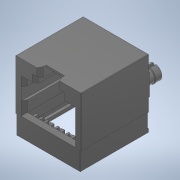
# Autodesk Inventor part: RJ45 Main Insert
Saved by Autodesk Inventor 2020.1 (Build 241239000, 239)
## iProperties
Created: 2019-12-05
Part Number: RJ45 Main Insert
Material: PBT Plastic
Document SubType Name: Modeling
Designer: S. Lee
Mass: 2.00676 g
Surface Area: 24.163 cm^2
Volume: 1.53188 cm^3
Density: 1.31 g/cm^3
Appearance: Smooth - Black
Author: S. Lee
Autodesk Inventor part; units mm, degrees
ref_plane "YZ Plane" through (0, 0, 0) normal (1, 0, 0) x (0, 1, 0)
ref_plane "XZ Plane" through (0, 0, 0) normal (0, 1, 0) x (-1, 0, 0)
ref_plane "XY Plane" through (0, 0, 0) normal (0, 0, 1) x (1, 0, 0)
sketch "Sketch1" plane through (0, 0, 0) normal (0, 0, 1) x (1, 0, 0)
  line L0 (-7.75, 8.125) -> (7.75, 8.125)
  line L1 (7.75, 8.125) -> (7.75, -3.775)
  line L2 (7.54, -8.125) -> (-7.54, -8.125)
  line L3 (-7.75, -3.775) -> (-7.75, 8.125)
  line L4 (-7.75, -3.775) -> (-7.54, -3.775)
  line L5 (-7.54, -3.775) -> (-7.54, -8.125)
  line L6 (7.75, -3.775) -> (7.54, -3.775)
  line L7 (7.54, -3.775) -> (7.54, -8.125)
  line L8 (0, -11.375) -> (0, 11.375) construction
  line L9 (-10.85, 0) -> (10.85, 0) construction
  dimension "d5" = 16.25
  dimension "d6" = 15.5
  dimension "d7" = 15.08
  dimension "d8" = 4.35
  constraints: 16 end point, 3 horizontal, 3 perpendicular, 2 parallel, 1 point on line, 3 other
  measures "d5" distance between parallel lines of L2 L0
  measures "d6" distance between parallel lines of L1 L3
  measures "d7" distance between parallel lines of L7 L5
  measures "d8" distance between parallel lines of L2 L4
extrude "Extrusion1" add sketch "Sketch1" against normal blind 16
sketch "Sketch2" plane through (0, 0, 0) normal (0, 0, 1) x (1, 0, 0)
  line L0 (5.925, -3.125) -> (-5.925, -3.125)
  line L1 (3.32, 4.125) -> (3.32, 5.825)
  line L2 (3.32, 5.825) -> (-3.32, 5.825)
  line L3 (-3.32, 5.825) -> (-3.32, 4.125)
  line L4 (-5.925, 4.125) -> (-3.32, 4.125)
  line L5 (3.32, 4.125) -> (5.925, 4.125)
  line L6 (-5.925, 2.325) -> (-6.425, 2.325)
  line L7 (-6.425, 2.325) -> (-6.425, -0.525)
  line L8 (-6.425, -0.525) -> (-5.925, -0.525)
  line L9 (5.925, 2.325) -> (6.425, 2.325)
  line L10 (6.425, 2.325) -> (6.425, -0.525)
  line L11 (6.425, -0.525) -> (5.925, -0.525)
  line L12 (-5.925, -3.125) -> (-5.925, -0.525)
  line L13 (-5.925, 2.325) -> (-5.925, 4.125)
  line L14 (5.925, 4.125) -> (5.925, 2.325)
  line L15 (5.925, -0.525) -> (5.925, -3.125)
  line L16 (0, -11.375) -> (0, 11.375) construction
  line L17 (-7.54, -8.125) -> (7.54, -8.125) construction
  point P0 (0, 0)
  dimension "d12" = 6.64
  dimension "d13" = 12.85
  dimension "d14" = 11.85
  dimension "d15" = 7.25
  dimension "d16" = 2.85
  dimension "d17" = 2.6
  dimension "d18" = 8.95
  dimension "d19" = 5
  constraints: 32 end point, 9 parallel, 6 perpendicular, 4 horizontal, 3 collinear, 2 point on line, 3 other
  measures "d12" distance between parallel lines of L1 L3
  measures "d13" distance between parallel lines of L10 L7
  measures "d14" distance between parallel lines of L15 L12
  measures "d15" distance between parallel lines of L0 L4
  measures "d16" distance between parallel lines of L8 L6
  measures "d17" distance between parallel lines of L0 L8
  measures "d18" distance between parallel lines of L0 L2
  measures "d19" distance between parallel lines of L17 L0
extrude "Extrusion2" cut sketch "Sketch2" against normal blind 12.7
sketch "Sketch3" plane through (0, 0, 0) normal (0, 0, 1) x (1, 0, 0)
  line L0 (-7.75, 8.125) -> (7.75, 8.125) construction
  line L1 (-3.32, 5.825) -> (3.32, 5.825) construction
  line L2 (-2.18, 8.125) -> (2.18, 8.125)
  line L3 (2.18, 8.125) -> (2.18, 5.825)
  line L4 (2.18, 5.825) -> (-2.18, 5.825)
  line L5 (-2.18, 5.825) -> (-2.18, 8.125)
  line L6 (0, -11.375) -> (0, 11.375) construction
  point P0 (0, 0)
  dimension "d22" = 4.36
  constraints: 8 end point, 2 parallel, 2 point on line, 1 horizontal, 1 perpendicular, 1 other
  measures "d22" distance of L3.end L4.end
extrude "Extrusion3" cut sketch "Sketch3" against normal blind 1.65
chamfer "Chamfer1" distance 0.5 distance2 1 1 edges at (0, -3.125, 0) measured on face at (0, -3.625, 0)
chamfer "Chamfer2" distance 0.5 distance2 1 2 edges at (-5.925, -3.375, 0) (-5.925, -1.825, 0) measured on face at (-6.425, -1.825, 0) measured on face at (-6.425, -3.375, 0)
chamfer "Chamfer3" distance 0.5 distance2 1 1 edges at (-5.925, 3.225, 0) measured on face at (-6.425, 3.225, 0)
chamfer "Chamfer4" distance 0.5 distance2 1 2 edges at (-6.175, 4.125, 0) (-4.6225, 4.125, 0) measured on face at (-4.6225, 4.625, 0) measured on face at (-6.175, 4.625, 0)
chamfer "Chamfer5" distance 0.5 distance2 1 1 edges at (-3.32, 5.225, 0) measured on face at (-3.82, 5.225, 0)
chamfer "Chamfer6" distance 0.5 distance2 1 2 edges at (-3.57, 5.825, 0) (-2.75, 5.825, 0) measured on face at (-2.75, 6.325, 0) measured on face at (-3.57, 6.325, 0)
chamfer "Chamfer7" distance 0.5 distance2 1 1 edges at (-2.18, 7.225, 0) measured on face at (-2.68, 7.225, 0)
chamfer "Chamfer8" distance 0.5 distance2 1 1 edges at (2.18, 6.975, 0) measured on face at (2.68, 6.975, 0)
chamfer "Chamfer9" distance 0.5 distance2 1 1 edges at (3, 5.825, 0)
chamfer "Chamfer10" distance 0.5 distance2 1 2 edges at (3.32, 6.0749, 0) (3.32, 4.975, 0) measured on face at (3.82, 6.0749, 0) measured on face at (3.82, 4.975, 0)
chamfer "Chamfer11" distance 0.5 distance2 1 1 edges at (4.8725, 4.125, 0) measured on face at (4.8725, 4.625, 0)
chamfer "Chamfer12" distance 0.5 distance2 1 2 edges at (5.925, 4.375, 0) (5.925, 3.225, 0) measured on face at (6.425, 3.225, 0) measured on face at (6.425, 4.375, 0)
chamfer "Chamfer13" distance 0.5 distance2 1 2 edges at (5.925, -1.825, 0) (5.925, -3.375, 0) measured on face at (6.425, -3.375, 0) measured on face at (6.425, -1.825, 0)
sketch "Sketch4" plane through (0, 0, -1.65) normal (0, 0, 1) x (1, 0, 0)
  line L0 (2.18, 5.825) -> (-2.18, 5.825) construction
  line L1 (-2.18, 7.695) -> (2.18, 7.695)
  line L2 (2.18, 7.695) -> (2.18, 5.825)
  line L3 (2.18, 5.825) -> (-2.18, 5.825)
  line L4 (-2.18, 5.825) -> (-2.18, 7.695)
  line L5 (-2.18, 5.825) -> (-2.18, 8.125) construction
  line L6 (2.18, 8.125) -> (2.18, 5.825) construction
  point P0 (0, 0)
  dimension "d64" = 1.87
  constraints: 8 end point, 2 collinear, 2 parallel, 1 horizontal, 1 perpendicular, 1 point on line
  measures "d64" distance between parallel lines of L0 L1
extrude "Extrusion4" cut sketch "Sketch4" against normal blind 1
sketch "Sketch5" plane through (0, 0, -2.65) normal (0, 0, 1) x (1, 0, 0)
  line L0 (2.18, 5.825) -> (-2.18, 5.825) construction
  line L1 (-2.18, 5.825) -> (2.18, 5.825)
  line L2 (2.18, 5.825) -> (2.18, 7.375)
  line L3 (2.18, 7.375) -> (-2.18, 7.375)
  line L4 (-2.18, 7.375) -> (-2.18, 5.825)
  line L5 (-2.18, 5.825) -> (-2.18, 7.695) construction
  line L6 (2.18, 7.695) -> (2.18, 5.825) construction
  point P0 (0, 0)
  dimension "d67" = 1.55
  constraints: 8 end point, 2 collinear, 2 parallel, 1 horizontal, 1 perpendicular, 1 point on line
  measures "d67" distance of L2.end L1.end
extrude "Extrusion5" cut sketch "Sketch5" against normal blind 3
chamfer "Chamfer14" distance 0.32 distance2 0.95 1 edges at (0, 7.375, -2.65) measured on face at (0, 7.475, -2.65)
sketch "Sketch6" plane through (0, 0, -16) normal (0, 0, -1) x (-1, 0, 0)
  line L0 (3.99, 7.025) -> (3.99, -0.65)
  line L1 (-3.99, -0.65) -> (-3.99, 7.025)
  line L2 (6.425, -8.125) -> (-6.425, -8.125)
  line L3 (-6.425, -0.65) -> (-3.99, -0.65)
  line L4 (3.99, -0.65) -> (6.425, -0.65)
  line L5 (0, -11.375) -> (0, 11.375) construction
  line L6 (7.75, 8.125) -> (-7.75, 8.125) construction
  line L7 (3.99, 7.025) -> (-3.99, 7.025)
  line L8 (-6.425, -5.925) -> (-7.06, -5.925)
  line L9 (-7.06, -5.925) -> (-7.06, -7.325)
  line L10 (-7.06, -7.325) -> (-6.425, -7.325)
  line L11 (6.425, -5.925) -> (7.06, -5.925)
  line L12 (7.06, -5.925) -> (7.06, -7.325)
  line L13 (7.06, -7.325) -> (6.425, -7.325)
  line L14 (-6.425, -8.125) -> (-6.425, -7.325)
  line L15 (-6.425, -5.925) -> (-6.425, -0.65)
  line L16 (6.425, -0.65) -> (6.425, -5.925)
  line L17 (6.425, -7.325) -> (6.425, -8.125)
  line L18 (-7.54, -8.125) -> (7.54, -8.125) construction
  point P0 (0, 0)
  dimension "d75" = 7.98
  dimension "d81" = 12.85
  dimension "d82" = 14.12
  dimension "d83" = 1.4
  dimension "d84" = 0.8
  dimension "d85" = 7.675
  dimension "d86" = 1.1
  constraints: 32 end point, 9 parallel, 6 perpendicular, 4 collinear, 4 horizontal, 2 point on line, 3 other
  measures "d75" distance between parallel lines of L0 L1
  measures "d81" distance between parallel lines of L16 L15
  measures "d82" distance between parallel lines of L12 L9
  measures "d83" distance between parallel lines of L10 L8
  measures "d84" distance between parallel lines of L2 L10
  measures "d85" distance between parallel lines of L3 L7
  measures "d86" distance between parallel lines of L6 L7
extrude "Extrusion6" cut sketch "Sketch6" against normal blind 1.2
sketch "Sketch8" plane through (0, 0, -14.8) normal (0, 0, -1) x (-1, 0, 0)
  line L0 (6.425, -8.125) -> (-6.425, -8.125) projected
  line L1 (-6.425, -8.125) -> (-6.425, -7.325) projected
  line L2 (-7.06, -7.325) -> (-7.06, -5.925) projected
  line L3 (-6.425, -5.925) -> (-6.425, -0.65) projected
  line L4 (-7.06, -5.925) -> (-6.425, -5.925) projected
  line L5 (6.425, -5.925) -> (7.06, -5.925) projected
  line L6 (6.425, -0.65) -> (6.425, -5.925) projected
  line L7 (7.06, -5.925) -> (7.06, -7.325) projected
  line L8 (6.425, -7.325) -> (6.425, -8.125) projected
  line L9 (-6.425, -7.325) -> (-7.06, -7.325) projected
  line L10 (7.06, -7.325) -> (6.425, -7.325) projected
  line L11 (-6.425, -3.125) -> (6.425, -3.125)
  point P0 (0, 0)
  dimension "d87" = 5
  constraints: 2 end point, 2 point on line, 1 perpendicular
  measures "d87" distance between parallel lines of L0 L11
extrude "Extrusion7" cut sketch "Sketch8" against normal blind 10.9
sketch "Sketch9" plane through (0, 0, -3.9) normal (0, 0, -1) x (-1, 0, 0)
  line L0 (-5.925, -3.125) -> (5.925, -3.125) projected
  line L1 (-7.06, -5.925) -> (-6.425, -5.925) projected
  line L2 (-7.06, -7.325) -> (-7.06, -5.925) projected
  line L3 (-6.425, -7.325) -> (-7.06, -7.325) projected
  line L4 (-6.425, -8.125) -> (-6.425, -7.325) projected
  line L5 (6.425, -8.125) -> (-6.425, -8.125) projected
  line L6 (6.425, -7.325) -> (6.425, -8.125) projected
  line L7 (7.06, -7.325) -> (6.425, -7.325) projected
  line L8 (7.06, -5.925) -> (7.06, -7.325) projected
  line L9 (6.425, -5.925) -> (7.06, -5.925) projected
  line L10 (6.425, -3.125) -> (6.425, -5.925) projected
  line L11 (5.925, -3.125) -> (6.425, -3.125) projected
  line L12 (-5.925, -3.125) -> (5.925, -3.125) projected
  line L13 (-6.425, -3.125) -> (-5.925, -3.125) projected
  line L14 (-6.425, -5.925) -> (-6.425, -3.125) projected
  line L15 (-6.425, -7.325) -> (6.425, -7.325)
  point P0 (0, 0)
  point P1 (5.925, -3.125)
  constraints: 2 end point, 1 horizontal
extrude "Extrusion8" cut sketch "Sketch9" against normal blind 2.9 contours L0 L11 L10 L9 L8 L7 L15 L3 L2 L1 L14 L13
sketch "Sketch10" plane through (0, 0, -14.8) normal (0, 0, -1) x (-1, 0, 0)
  line L0 (-3.99, 7.025) -> (3.99, 7.025) projected
  line L1 (3.99, 7.025) -> (3.99, -0.65) projected
  line L2 (-3.99, 7.025) -> (3.99, 7.025)
  line L3 (3.99, 7.025) -> (3.99, 5.825)
  line L4 (3.99, 5.825) -> (-3.99, 5.825)
  line L5 (-3.99, 5.825) -> (-3.99, 7.025)
  point P0 (0, 0)
  dimension "d92" = 1.2
  constraints: 8 end point, 2 parallel, 1 horizontal, 1 perpendicular, 1 point on line
  measures "d92" distance between parallel lines of L4 L0
extrude "Extrusion9" cut sketch "Sketch10" against normal blind 11.2
sketch "Sketch11" plane through (0, 0, -12.7) normal (0, 0, 1) x (1, 0, 0)
  line L0 (6.425, -3.125) -> (-6.425, -3.125) projected
  line L1 (-4.67, -3.125) -> (-4.22, -3.125)
  line L2 (-4.22, -3.125) -> (-4.22, 1.225)
  line L3 (-4.22, 1.225) -> (-4.67, 1.225)
  line L4 (-4.67, 1.225) -> (-4.67, -3.125)
  line L5 (-7.75, -3.775) -> (-7.75, 8.125) projected
  line L6 (-3.4, -3.125) -> (-2.95, -3.125)
  line L7 (-2.95, -3.125) -> (-2.95, 1.225)
  line L8 (-2.95, 1.225) -> (-3.4, 1.225)
  line L9 (-3.4, 1.225) -> (-3.4, -3.125)
  line L10 (-2.13, -3.125) -> (-1.68, -3.125)
  line L11 (-1.68, -3.125) -> (-1.68, 1.225)
  line L12 (-1.68, 1.225) -> (-2.13, 1.225)
  line L13 (-2.13, 1.225) -> (-2.13, -3.125)
  line L14 (-0.86, -3.125) -> (-0.41, -3.125)
  line L15 (-0.41, -3.125) -> (-0.41, 1.225)
  line L16 (-0.41, 1.225) -> (-0.86, 1.225)
  line L17 (-0.86, 1.225) -> (-0.86, -3.125)
  line L18 (0.41, -3.125) -> (0.86, -3.125)
  line L19 (0.86, -3.125) -> (0.86, 1.225)
  line L20 (0.86, 1.225) -> (0.41, 1.225)
  line L21 (0.41, 1.225) -> (0.41, -3.125)
  line L22 (1.68, -3.125) -> (2.13, -3.125)
  line L23 (2.13, -3.125) -> (2.13, 1.225)
  line L24 (2.13, 1.225) -> (1.68, 1.225)
  line L25 (1.68, 1.225) -> (1.68, -3.125)
  line L26 (2.95, -3.125) -> (3.4, -3.125)
  line L27 (3.4, -3.125) -> (3.4, 1.225)
  line L28 (3.4, 1.225) -> (2.95, 1.225)
  line L29 (2.95, 1.225) -> (2.95, -3.125)
  line L30 (4.22, -3.125) -> (4.67, -3.125)
  line L31 (4.67, -3.125) -> (4.67, 1.225)
  line L32 (4.67, 1.225) -> (4.22, 1.225)
  line L33 (4.22, 1.225) -> (4.22, -3.125)
  point P0 (0, 0)
  dimension "d95" = 0.45
  dimension "d96" = 4.35
  dimension "d97" = 3.08
  dimension "d100" = 1.27
  constraints: 64 end point, 2 horizontal, 2 parallel, 1 perpendicular, 1 point on line, 56 other
  measures "d95" distance of L3.end L2.end
  measures "d96" distance of L1.end L2.end
  measures "d97" distance between parallel lines of L5 L4
  measures "d100" distance of L1.start L6.start
extrude "Extrusion10" cut sketch "Sketch11" against normal up to surface (2.1 mm away)
chamfer "Chamfer15" distance 0.9 distance2 2.1 1 edges at (3.81, -3.125, -14.8) measured on face at (3.81, -2.625, -14.8)
chamfer "Chamfer16" distance 0.9 distance2 2.1 1 edges at (2.54, -3.125, -14.8) measured on face at (2.54, -2.625, -14.8)
chamfer "Chamfer17" distance 0.9 distance2 2.1 1 edges at (1.27, -3.125, -14.8) measured on face at (1.27, -2.625, -14.8)
chamfer "Chamfer18" distance 0.9 distance2 2.1 1 edges at (0, -3.125, -14.8) measured on face at (0, -2.625, -14.8)
chamfer "Chamfer19" distance 0.9 distance2 2.1 1 edges at (-1.27, -3.125, -14.8) measured on face at (-1.27, -2.625, -14.8)
chamfer "Chamfer20" distance 0.9 distance2 2.1 1 edges at (-2.54, -3.125, -14.8) measured on face at (-2.54, -2.625, -14.8)
chamfer "Chamfer21" distance 0.9 distance2 2.1 1 edges at (-3.81, -3.125, -14.8) measured on face at (-3.81, -2.625, -14.8)
chamfer "Chamfer22" distance 0.9 distance2 2.1 1 edges at (1.905, 1.225, -14.8) measured on face at (1.905, 1.725, -14.8)
chamfer "Chamfer23" distance 0.9 distance2 2.1 1 edges at (3.175, 1.225, -14.8) measured on face at (3.175, 1.725, -14.8)
chamfer "Chamfer24" distance 0.9 distance2 2.1 1 edges at (0.635, 1.225, -14.8) measured on face at (0.635, 1.725, -14.8)
chamfer "Chamfer25" distance 0.9 distance2 2.1 1 edges at (-0.635, 1.225, -14.8) measured on face at (-0.635, 1.725, -14.8)
chamfer "Chamfer26" distance 0.9 distance2 2.1 1 edges at (-1.905, 1.225, -14.8) measured on face at (-1.905, 1.725, -14.8)
chamfer "Chamfer27" distance 0.9 distance2 2.1 1 edges at (-3.175, 1.225, -14.8) measured on face at (-3.175, 1.725, -14.8)
sketch "Sketch12" plane through (-4.67, -3.125, -12.7) normal (1, 0, 0) x (0, 0, -1)
  line L0 (0, 4.35) -> (2.1, 5.25) projected
  line L1 (2.1, 5.25) -> (2.1, 2.475)
  line L2 (2.1, 2.475) -> (0, 2.475)
  line L3 (0, 2.475) -> (0, 4.35)
  line L4 (3.3, 2.475) -> (2.1, 2.475) construction
  point P0 (-12.7, 3.125)
  constraints: 6 end point, 2 perpendicular, 1 collinear, 1 vertical
extrude "Extrusion11" cut sketch "Sketch12" along normal up to surface (0.45 mm away)
sketch "Sketch13" plane through (4.22, -0.65, -14.8) normal (1, 0, 0) x (0, 0, -1)
  line L0 (-2.1, 1.875) -> (0, 2.775) projected
  line L1 (1.2, 0) -> (0, 0) projected
  line L2 (0, 2.775) -> (0, 0)
  line L3 (0, 0) -> (-2.1, 0)
  line L4 (-2.1, 1.875) -> (-2.1, -2.475) projected
  line L5 (-2.1, 0) -> (-2.1, 1.875)
  point P0 (-14.8, 0.65)
  constraints: 6 end point, 2 perpendicular, 1 collinear
extrude "Extrusion12" cut sketch "Sketch13" along normal up to surface (0.45 mm away)
sketch "Sketch14" plane through (0, 0, -16) normal (0, 0, -1) x (-1, 0, 0)
  line L0 (-7.75, -3.775) -> (-7.75, 8.125) construction
  line L1 (-7.75, 4.3) -> (-5.85, 4.3)
  line L2 (-5.85, 4.3) -> (-5.85, -0.65)
  line L3 (-5.85, -0.65) -> (-7.75, -0.65)
  line L4 (-7.75, -0.65) -> (-7.75, 4.3)
  line L5 (-6.425, -0.65) -> (-3.99, -0.65) construction
  arc A0 (-5.85, 0.2558) -> (-5.85, 3.3942) centre (-5.715, 1.825) ccw
  point P0 (0, 0)
  dimension "d150" = 1.9
  dimension "d151" = 4.95
  dimension "d154" = 2.475
  dimension "d157" = 1.575
  dimension "d158" = 2.035
  constraints: 6 end point, 2 horizontal, 2 point on circle, 1 centre point, 1 collinear, 1 parallel, 1 point on line, 1 vertical, 5 other
  measures "d150" distance of L3.start L3.end
  measures "d151" distance of L1.end L3.start
  measures "d154" distance from line of L1 A0.centre
  measures "d157" radius of A0
  measures "d158" distance from line of L0 A0.centre
extrude "Extrusion13" add sketch "Sketch14" along normal blind 0.2
sketch "Sketch15" plane through (0, 0, -16.2) normal (0, 0, -1) x (-1, 0, 0)
  arc A0 (-5.85, 0.2558) -> (-5.85, 3.3942) centre (-5.715, 1.825) ccw projected
  circle A1 centre (-5.715, 1.825) radius 1.575
  line L0 (-6.065, 3.3606) -> (-6.065, 0.2894)
  line L1 (-5.365, 0.2894) -> (-5.365, 3.3606)
  line L2 (-5.715, 1.825) -> (-5.715, 3.4) construction
  point P0 (0, 0)
  dimension "d159" = 0.7
  constraints: 6 end point, 5 point on circle, 2 vertical, 1 centre point, 1 coincident, 1 concentric, 1 parallel, 1 other
  measures "d159" distance between parallel lines of L1 L0
extrude "Extrusion14" add sketch "Sketch15" along normal blind 1.65 contours L1 A0 | A1 L0
sketch "Sketch16" plane through (0, 0, -17.85) normal (0, 0, -1) x (-1, 0, 0)
  line L0 (-5.365, 3.3606) -> (-5.365, 0.2894) construction
  line L1 (-6.065, 0.2894) -> (-6.065, 3.3606) construction
  circle A0 centre (-5.715, 1.825) radius 1.725
  line L2 (-6.065, 3.5141) -> (-6.065, 0.1359)
  line L3 (-5.365, 3.5141) -> (-5.365, 0.1359)
  arc A1 (-6.065, 3.3606) -> (-6.065, 0.2894) centre (-5.715, 1.825) ccw projected
  point P0 (0, 0)
  dimension "d162" = 3.45
  constraints: 4 end point, 4 point on circle, 2 collinear, 1 centre point, 1 coincident, 1 vertical
  measures "d162" diameter of A0
extrude "Extrusion15" add sketch "Sketch16" along normal blind 1.85 contours A0 L3 | L2 A1 A0 | L2 A1
chamfer "Chamfer28" distance 0.15 angle 45 2 edges at (7.44, 1.825, -17.85) (3.99, 1.825, -17.85)
chamfer "Chamfer29" distance 0.6 distance2 0.3 1 edges at (7.44, 1.825, -19.7) measured on face at (6.94, 1.825, -19.7)
chamfer "Chamfer30" distance 0.6 distance2 0.3 1 edges at (3.99, 1.825, -19.7) measured on face at (4.49, 1.825, -19.7)
sketch "Sketch17" plane through (0, 0, -16) normal (0, 0, -1) x (-1, 0, 0)
  circle A0 centre (-6.3, 6.975) radius 0.45
  line L0 (7.75, 8.125) -> (-7.75, 8.125) construction
  line L1 (-7.75, 8.125) -> (-7.75, 4.3) construction
  line L2 (-6.425, -8.125) -> (-6.425, -7.325) projected
  line L3 (-7.54, -3.775) -> (-7.54, -8.125) projected
  line L4 (-6.425, -7.325) -> (-7.54, -7.325)
  line L5 (-7.54, -7.325) -> (-7.54, -8.125)
  line L6 (-7.54, -8.125) -> (-6.425, -8.125)
  line L7 (-6.425, -8.125) -> (-6.425, -7.325)
  point P0 (0, 0)
  dimension "d174" = 0.9
  dimension "d175" = 1.15
  dimension "d176" = 1.45
  constraints: 8 end point, 2 parallel, 1 centre point, 1 horizontal, 1 perpendicular
  measures "d174" diameter of A0
  measures "d175" distance from line of L0 A0.centre
  measures "d176" distance from line of L1 A0.centre
extrude "Extrusion16" add sketch "Sketch17" along normal blind 0.2
mirror "Mirror1" about plane through (0, 0, 0) normal (1, 0, 0) of "Extrusion16", "Extrusion15", "Extrusion14", "Extrusion13", "Chamfer28", "Chamfer29", "Chamfer30"
sketch "Sketch19" plane through (0, 0, -1) normal (0, 0, -1) x (-1, 0, 0)
  line L0 (6.425, -7.325) -> (-6.425, -7.325) construction
  line L1 (-6.425, -8.125) -> (-6.425, -7.325) construction
  line L2 (6.425, -8.125) -> (-6.425, -8.125) construction
  line L3 (6.425, -7.325) -> (6.425, -8.125) construction
  line L4 (-4.67, 1.225) -> (-4.67, -3.125) construction
  line L5 (-4.22, -3.125) -> (-4.22, 1.225) construction
  line L6 (-4.22, -7.325) -> (4.22, -7.325)
  line L7 (4.22, -7.325) -> (4.22, -5.825)
  line L8 (4.22, -5.825) -> (-4.22, -5.825)
  line L9 (-4.22, -5.825) -> (-4.22, -7.325)
  line L10 (-4.67, -3.125) -> (-4.22, -3.125)
  line L11 (-4.22, -3.125) -> (-4.22, -5.125)
  line L12 (-4.22, -5.125) -> (-4.67, -5.125)
  line L13 (-4.67, -5.125) -> (-4.67, -3.125)
  line L14 (0, -11.375) -> (0, 11.375) construction
  line L15 (-3.4, -3.125) -> (-2.95, -3.125)
  line L16 (-2.95, -3.125) -> (-2.95, -5.125)
  line L17 (-2.95, -5.125) -> (-3.4, -5.125)
  line L18 (-3.4, -5.125) -> (-3.4, -3.125)
  line L19 (-2.13, -3.125) -> (-1.68, -3.125)
  line L20 (-1.68, -3.125) -> (-1.68, -5.125)
  line L21 (-1.68, -5.125) -> (-2.13, -5.125)
  line L22 (-2.13, -5.125) -> (-2.13, -3.125)
  line L23 (-0.86, -3.125) -> (-0.41, -3.125)
  line L24 (-0.41, -3.125) -> (-0.41, -5.125)
  line L25 (-0.41, -5.125) -> (-0.86, -5.125)
  line L26 (-0.86, -5.125) -> (-0.86, -3.125)
  line L27 (0.41, -3.125) -> (0.86, -3.125)
  line L28 (0.86, -3.125) -> (0.86, -5.125)
  line L29 (0.86, -5.125) -> (0.41, -5.125)
  line L30 (0.41, -5.125) -> (0.41, -3.125)
  line L31 (1.68, -3.125) -> (2.13, -3.125)
  line L32 (2.13, -3.125) -> (2.13, -5.125)
  line L33 (2.13, -5.125) -> (1.68, -5.125)
  line L34 (1.68, -5.125) -> (1.68, -3.125)
  line L35 (2.95, -3.125) -> (3.4, -3.125)
  line L36 (3.4, -3.125) -> (3.4, -5.125)
  line L37 (3.4, -5.125) -> (2.95, -5.125)
  line L38 (2.95, -5.125) -> (2.95, -3.125)
  line L39 (4.22, -3.125) -> (4.67, -3.125)
  line L40 (4.67, -3.125) -> (4.67, -5.125)
  line L41 (4.67, -5.125) -> (4.22, -5.125)
  line L42 (4.22, -5.125) -> (4.22, -3.125)
  point P0 (0, 0)
  dimension "d179" = 1.5
  dimension "d180" = 8.44
  dimension "d181" = 2
  dimension "d184" = 1.27
  constraints: 72 end point, 4 parallel, 3 horizontal, 2 perpendicular, 1 collinear, 1 point on line, 57 other
  measures "d179" distance of L8.end L6.start
  measures "d180" distance between parallel lines of L7 L9
  measures "d181" distance between parallel lines of L12 L10
  measures "d184" distance of L4.end L15.start
extrude "Extrusion17" add sketch "Sketch19" along normal blind 0.8
sketch "Sketch20" plane through (0, 0, -1) normal (0, 0, -1) x (-1, 0, 0)
  line L0 (-4.67, -5.25) -> (-4.22, -5.25)
  line L1 (-4.22, -5.25) -> (-4.22, -5.7)
  line L2 (-4.22, -5.7) -> (-4.67, -5.7)
  line L3 (-4.67, -5.7) -> (-4.67, -5.25)
  line L4 (-2.13, -5.25) -> (-1.68, -5.25)
  line L5 (-1.68, -5.25) -> (-1.68, -5.7)
  line L6 (-1.68, -5.7) -> (-2.13, -5.7)
  line L7 (-2.13, -5.7) -> (-2.13, -5.25)
  line L8 (0.41, -5.25) -> (0.86, -5.25)
  line L9 (0.86, -5.25) -> (0.86, -5.7)
  line L10 (0.86, -5.7) -> (0.41, -5.7)
  line L11 (0.41, -5.7) -> (0.41, -5.25)
  line L12 (2.95, -5.25) -> (3.4, -5.25)
  line L13 (3.4, -5.25) -> (3.4, -5.7)
  line L14 (3.4, -5.7) -> (2.95, -5.7)
  line L15 (2.95, -5.7) -> (2.95, -5.25)
  line L16 (-4.22, -5.125) -> (-4.67, -5.125) projected
  line L17 (-4.22, -3.125) -> (-4.22, -5.125) projected
  line L18 (4.67, -5.7) -> (4.67, -5.25)
  line L19 (4.67, -5.25) -> (5.12, -5.25)
  line L20 (5.12, -5.25) -> (5.12, -5.7)
  line L21 (5.12, -5.7) -> (4.67, -5.7)
  point P0 (0, 0)
  dimension "d198" = 10
  dimension "d191" = 0.45
  dimension "d192" = 0.45
  dimension "d195" = 2.54
  dimension "d200" = 0.125
  dimension "d203" = 1.72
  constraints: 40 end point, 3 collinear, 3 horizontal, 2 parallel, 1 perpendicular, 30 other
  measures "d191" distance of L1.end L2.end
  measures "d192" distance of L0.end L1.end
  measures "d195" distance of L0.start L4.start
  measures "d200" distance between parallel lines of L0 L16
  measures "d203" distance of L12.start L18.end
extrude "Extrusion18" add sketch "Sketch20" along normal blind 2.9
fillet "Fillet1" radius 0.1 31 edges at (7.54, -5.55, -16) (7.54, -7.325, -16.1) (7.54, -8.125, -8) (7.54, -8.125, -16.1) (7.54, -7.725, -16.2) (6.9825, -8.125, -16.2) (7.54, -3.775, -8) (7.75, -3.775, -8) (7.645, -3.775, -16) (7.75, -2.2125, -16) (7.75, 6.2125, -16) (7.75, 8.125, -8) (0, 8.125, -16) (7.75, 2.175, 0) (7.54, -5.95, 0) (7.645, -3.775, 0) (0, -8.125, 0) (-7.54, -5.95, 0) (-7.645, -3.775, 0) (-7.75, -3.775, -8) (-7.75, 2.175, 0) (-7.75, 8.125, -8) (-7.75, 6.2125, -16) (-7.54, -8.125, -8) (-7.54, -8.125, -16.1) (-6.9825, -8.125, -16.2) (-7.54, -7.725, -16.2) (-7.54, -7.325, -16.1) (-7.54, -5.55, -16) (-7.75, -2.2125, -16) (-7.645, -3.775, -16)
chamfer "Chamfer31" distance 0.05 angle 45 20 edges at (4.445, -5.7, -3.9) (4.22, -5.475, -3.9) (4.445, -5.25, -3.9) (4.67, -5.475, -3.9) (2.13, -5.475, -3.9) (1.905, -5.7, -3.9) (1.68, -5.475, -3.9) (1.905, -5.25, -3.9) (-0.635, -5.7, -3.9) (-0.41, -5.475, -3.9) (-0.635, -5.25, -3.9) (-0.86, -5.475, -3.9) (-3.175, -5.7, -3.9) (-3.4, -5.475, -3.9) (-3.175, -5.25, -3.9) (-2.95, -5.475, -3.9) (-4.67, -5.475, -3.9) (-4.895, -5.25, -3.9) (-5.12, -5.475, -3.9) (-4.895, -5.7, -3.9)
ref_plane "Work Plane1" through (0, 0, 0) normal (1, 0, 0) x (0, 1, 0)
equation "\"d154\" = 0.5 * d151"
body "Solid1"
